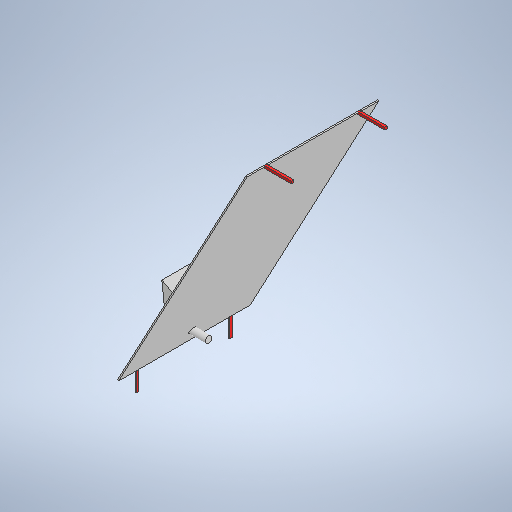
# Autodesk Inventor part: Pocket
Saved by Autodesk Inventor 2026.2 (Build 302298000, 298)
## iProperties
Created: 2026-07-16
Part Number: Pocket
Material: Generic
Document SubType Name: Modeling
Designer: admin
Density: 1 g/cm^3
Appearance: Default
Mass: 673442 g
Surface Area: 220356 cm^2
Volume: 673442 cm^3
allow_slope_adjustment: 0 ul
flow_configuration2: 1 ul
flow_direction: 2 ul
loss_method: 0 ul
radius: 55,000 mm
Author: admin
Autodesk Inventor part; units mm, degrees
ref_plane "YZ Plane" through (0, 0, 0) normal (1, 0, 0) x (0, 1, 0)
ref_plane "XZ Plane" through (0, 0, 0) normal (0, 1, 0) x (-1, 0, 0)
ref_plane "XY Plane" through (0, 0, 0) normal (0, 0, 1) x (1, 0, 0)
sketch "Sketch1" plane through (0, 0, 0) normal (0, 0, 1) x (1, 0, 0)
  line L0 (-440, 0) -> (-440, 4350)
  line L1 (-440, 4350) -> (-2590, 320)
  line L2 (-2590, 320) -> (-2590, 0)
  line L3 (-2590, 0) -> (-440, 0)
  line L4 (-2590, 320) -> (-2607.6458, 329.414)
  line L5 (-2607.6458, 329.414) -> (-457.6458, 4359.414)
  line L6 (-457.6458, 4359.414) -> (-440, 4350)
  point P0 (0, 0)
  dimension "d0" = 4350
  dimension "d1" = 2150
  dimension "d2" = 320
  dimension "d3" = 61.92
  dimension "d4" = 440
  dimension "d5" = 20
  constraints: 14 end point, 4 perpendicular, 1 horizontal alignment, 1 parallel, 1 vertical
  measures "d0" distance of L0.start L0.end
  measures "d1" distance of L2.end L0.start
  measures "d2" distance of L1.end L2.end
  measures "d3" angle of L3 L1
  measures "d4" distance from line of point (0, 0) L0
  measures "d5" distance of L5.end L0.end
extrude "Extrusion1" add sketch "Sketch1" along normal mid plane 2200 contours L1 L4 L5 L6
sketch "Sketch2" plane through (-2607.6458, 329.414, -1100) normal (-0.8822923, 0.4707019, 0) x (0, 0, 1)
  line L0 (0, 0) -> (0, 4567.6471) projected
  line L1 (0, 0) -> (2200, 0) projected
  line L2 (2200, 4567.6471) -> (2200, 0) projected
  line L3 (0, 4567.6471) -> (2200, 4567.6471) projected
  line L4 (0, 1950) -> (1000, 0)
  line L5 (2200, 1950) -> (1200, 0)
  line L6 (0, 1950) -> (2200, 1950)
  point P0 (1100, 936.7843)
  dimension "d8" = 1950
  dimension "d9" = 200
  constraints: 6 end point, 4 point on line, 1 equal length, 1 perpendicular
  measures "d8" distance between parallel lines of L1 L6
  measures "d9" distance of L5.end L4.end
extrude "Extrusion2" add sketch "Sketch2" along normal blind 200 contours L6 L5 L1 L4
sketch "Sketch3" plane through (0, 0, 0) normal (0, 0, 1) x (1, 0, 0)
  line L0 (-2590, 320) -> (-440, 4350) construction
  line L1 (-2483.3002, 575) -> (-2183.3002, 575)
  line L2 (-2483.3002, 575) -> (-2483.3002, 520)
  line L3 (-2483.3002, 520) -> (-2183.3002, 520)
  line L4 (-2183.3002, 520) -> (-2183.3002, 575)
  point P0 (0, 0)
  dimension "d12" = 300
  dimension "d13" = 200
  dimension "d14" = 110
  constraints: 8 end point, 2 perpendicular, 1 horizontal, 1 point on line, 1 vertical
  measures "d12" distance of L1.start L1.end
  measures "d13" distance from line of L0.start L3
  measures "d14" diameter of L3 L1
revolve "Revolution1" add sketch "Sketch3" angle 360 about axis through (-2483.3002, 575, 0) along (1, 0, 0)
sketch "Sketch4" plane through (0, 0, 0) normal (0, 1, 0) x (-1, 0, 0)
  line L0 (2607.6458, 100) -> (2607.6458, 1100) projected
  line L1 (2590, -1100) -> (2590, 1100) projected
  line L2 (2590, 800) -> (2607.6458, 800)
  line L3 (2607.6458, 800) -> (2607.6458, 760)
  line L4 (2607.6458, 760) -> (2590, 760)
  line L5 (2590, 760) -> (2590, 800)
  point P0 (0, 0)
  dimension "d16" = 40
  dimension "d17" = 300
  constraints: 8 end point, 2 parallel, 2 point on line, 1 horizontal, 1 perpendicular
  measures "d16" distance between parallel lines of L4 L2
  measures "d17" distance from line of L2 L0.end
extrude "Extrusion3" add sketch "Sketch4" along normal up to surface surface through (-457.6458, 4359.414, 0) normal (-0.8822923, 0.4707019, 0)
sketch "Sketch5" plane through (0, 0, 0) normal (1, 0, 0) x (0, 1, 0)
  line L0 (4359.414, -1100) -> (4359.414, 1100) projected
  line L1 (4359.414, 760) -> (4319.414, 760)
  line L2 (4319.414, 760) -> (4319.414, 800)
  line L3 (4319.414, 800) -> (4359.414, 800)
  line L4 (4359.414, 800) -> (4359.414, 760)
  point P0 (0, 0)
  dimension "d20" = 40
  dimension "d24" = 300
  constraints: 8 end point, 2 parallel, 2 perpendicular, 1 horizontal, 1 point on line
  measures "d20" distance of L2.end L3.end
  measures "d24" distance from line of L0.end L3
extrude "Extrusion4" add sketch "Sketch5" against normal up to surface surface through (-457.6458, 4359.414, 0) normal (-0.8822923, 0.4707019, 0)
mirror "Mirror2" about plane through (0, 0, 0) normal (0, 0, 1) of "Extrusion3", "Extrusion4"
body "Solid1"
